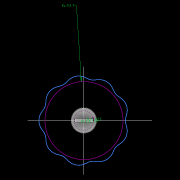
# Autodesk Inventor part: OuterRaceTool
Saved by Autodesk Inventor 2022.2 (Build 262287010, 287A)
## iProperties
Created: 2022-05-21
Part Number: OuterRaceTool
Material: Generic
Document SubType Name: Modeling
Designer: Árni Þór Þorgeirsson
Density: 1 g/cm^3
Appearance: Default
Author: Árni Þór Þorgeirsson
Autodesk Inventor part; units mm, degrees
ref_plane "YZ Plane" through (0, 0, 0) normal (1, 0, 0) x (0, 1, 0)
ref_plane "XZ Plane" through (0, 0, 0) normal (0, 1, 0) x (-1, 0, 0)
sketch "Sketch7" plane through (0, 0, 0) normal (0, 1, 0) x (-1, 0, 0)
  line L0 (0, 0) -> (0, 15.7673)
  line L1 (0, 0) -> (-13.3368, 0) construction
  line L2 (0, 15.7673) -> (-13.3368, 0) construction
  line L3 (0, 15.7673) -> (-18.6413, 0) construction
  line L4 (0, 15.7673) -> (-12.4569, -5.231) construction
  line L5 (0, 0) -> (0, -15.7673)
  line L6 (0, -15.7673) -> (-13.3368, 0) construction
  line L7 (0, -15.7673) -> (-18.6413, 0) construction
  line L8 (0, -15.7673) -> (-12.4569, 5.231) construction
  line L9 (-12.4569, 5.231) -> (-18.6413, 0) construction
  line L10 (-9.3537, 0) -> (-18.5948, -7.8164) construction
  line L11 (-9.3537, 0) -> (-18.0926, 7.3915) construction
  line L12 (0, -29.7093) -> (0, 66.7435) projected
  line L13 (-53.5, -5.9919) -> (-53.5, 6.008)
  line L14 (17.5786, 0) -> (-94.9714, 0) projected
  line L15 (-15.989, 2.2434) -> (-10.6846, -2.2434) construction
  line L16 (-10.6846, 2.2434) -> (-15.989, -2.2434) construction
  line L17 (-26.151, -15.9303) -> (-40.3783, -15.9303) construction
  line L18 (-40.3783, -15.9303) -> (-40.3783, -12.7539) construction
  line L19 (-40.3783, -12.7539) -> (-26.151, -12.7539) construction
  line L20 (-26.151, -12.7539) -> (-26.151, -15.9303) construction
  point P0 (-53.5, 0)
  dimension "Roller_Side_difference" = -0.0003
  dimension "d90" = 15.7673
  dimension "d201" = 53.5
  dimension "d343" = 99.548
  dimension "d344" = 99.549
  dimension "d367" = 8.1
  constraints: 28 end point, 9 point on line, 3 midpoint, 3 vertical, 2 horizontal, 2 parallel, 2 perpendicular, 1 collinear, 1 symmetric about line, 2 other
  measures "d90" distance of L0.start L0.end
  measures "d201" distance between parallel lines of L5 L13
  measures "d343" angle of L10 L8
  measures "d344" angle of L7 L10
  measures "d367" distance of L3.end L8.end
sketch "Sketch1" plane through (0, 0, 0) normal (0, 0, 1) x (1, 0, 0)
  circle A0 centre (0, 0) radius 13.3368 construction
  line L0 (0, 0) -> (13.3368, 0)
  line L1 (0, 0) -> (13.3368, 4.025)
  line L2 (13.3368, 0) -> (13.3368, 4.025)
  circle A1 centre (0, 0) radius 53.5
  point P0 (56.8, 0)
  dimension "d56" = 13.3368
  dimension "d57" = 4.025
  dimension "d400" = 53.5
  dimension "d495" = 2.5
  dimension "d496" = 8
  dimension "d531" = 5.5
  dimension "d532" = 5.5
  dimension "d533" = 5.5
  dimension "d537" = 24.5
  dimension "d538" = 3
  dimension "d543" = 5.5
  dimension "d549" = 3
  dimension "d550" = 3
  dimension "d567" = 5.5
  dimension "d568" = 5.5
  constraints: 1 other
sketch "Roller1" plane through (0, 0, 0) normal (0, 1, 0) x (-1, 0, 0)
  line L0 (0, 15.7673) -> (-12.4569, -5.231) construction
  line L1 (0, 15.7673) -> (-18.6413, 0) construction
  line L2 (-9.3537, 0) -> (-18.0926, 7.3915) construction
  line L3 (0, -15.7673) -> (-18.6413, 0) construction
  line L4 (-9.4248, -0.0708) -> (-12.4245, -5.1274)
  line L5 (-12.4245, -5.1274) -> (-18.5445, 0.0491)
  line L6 (-18.5445, 0.0491) -> (-14.0556, 3.846)
  line L7 (-14.0556, 3.846) -> (-9.4248, -0.0708)
  line L8 (-11.7456, 1.8921) -> (-15.4898, -2.5346)
  line L9 (-10.9821, 1.2463) -> (-14.7263, -3.1804)
  point P0 (0, 0)
  point P1 (-15.4845, -2.5391)
  dimension "d345" = 0.025
  dimension "d346" = 0.025
  dimension "d347" = 0.1
  dimension "d348" = 0.1
  dimension "d349" = 99.549
  dimension "d350" = 99.548
  dimension "d357" = 1
  dimension "d369" = 4.0148
  constraints: 12 end point, 5 parallel, 4 point on line, 1 midpoint, 1 perpendicular
  measures "d345" distance between parallel lines of L0 L4
  measures "d346" distance between parallel lines of L1 L6
  measures "d347" distance between parallel lines of L3 L5
  measures "d348" distance between parallel lines of L2 L7
  measures "d349" angle of L6 L7
  measures "d350" angle of L4 L7
  measures "d357" distance between parallel lines of L8 L9
  measures "d369" distance from line of L4.end L8
sketch "Roller2" plane through (0, 0, 0) normal (0, 1, 0) x (-1, 0, 0)
  line L0 (0, -15.7673) -> (-12.4569, 5.231) construction
  line L1 (-9.3537, 0) -> (-18.5948, -7.8164) construction
  line L2 (0, -15.7673) -> (-18.6413, 0) construction
  line L3 (0, 15.7673) -> (-18.6413, 0) construction
  line L4 (-12.4245, 5.1274) -> (-9.4248, 0.0708)
  line L5 (-9.4248, 0.0708) -> (-14.0556, -3.846)
  line L6 (-14.0556, -3.846) -> (-18.5445, -0.0491)
  line L7 (-18.5445, -0.0491) -> (-12.4245, 5.1274)
  line L8 (-15.4845, 2.5391) -> (-11.7403, -1.8876)
  line L9 (-14.721, 3.1849) -> (-10.9767, -1.2418)
  point P0 (0, 0)
  dimension "d351" = 0.025
  dimension "d352" = 0.025
  dimension "d354" = 0.1
  dimension "d355" = 99.548
  dimension "d356" = 99.549
  dimension "d370" = 0.1
  dimension "d371" = 1
  constraints: 12 end point, 5 parallel, 3 point on line, 1 midpoint, 1 perpendicular
  measures "d351" distance between parallel lines of L0 L4
  measures "d352" distance between parallel lines of L2 L6
  measures "d354" distance between parallel lines of L1 L5
  measures "d355" angle of L5 L4
  measures "d356" angle of L6 L5
  measures "d370" distance from line of L3 L8.start
  measures "d371" distance between parallel lines of L9 L8
sketch "Sketch22" plane through (0, 0, 0) normal (0, 1, 0) x (-1, 0, 0)
  line L0 (-31.756, 8.0215) -> (-17.5287, 8.0215) construction
  line L1 (-17.5287, 8.0215) -> (-17.5287, 4.8451) construction
  line L2 (-17.5287, 4.8451) -> (-31.756, 4.8451) construction
  line L3 (-31.756, 4.8451) -> (-31.756, 8.0215) construction
  point P0 (0, 0)
  dimension "Roller_Side_difference" = -0.0003
  constraints: 2 other
sketch "Sketch2" plane through (0, 0, 0) normal (0, 1, 0) x (-1, 0, 0)
  line L0 (0, 0) -> (0, 13.3368) construction
  line L1 (0, 0) -> (-13.3368, 0) projected
  line L2 (0, 0) -> (0, -13.3368)
  line L3 (0, -13.3368) -> (-13.3368, 0) construction
  line L4 (0, 13.3368) -> (-13.3368, 0) construction
  line L5 (-78.8928, 52.9645) -> (0, 13.3368) construction
  line L6 (-34.8011, 15.91) -> (0, 13.3368) construction
  line L7 (-34.8011, 15.91) -> (0, -13.3368) construction
  line L8 (-48.3339, 16.9106) -> (0, -13.3368) construction
  point P0 (-17.4708, -4.134)
  constraints: 16 end point, 3 point on line, 1 perpendicular, 1 symmetric about line, 1 vertical
sketch "Sketch23" plane through (0, 0, 0) normal (0, 1, 0) x (-1, 0, 0)
  line L0 (0, -15.7673) -> (-12.4569, 5.231) construction
  line L1 (0, -15.7673) -> (-18.6413, 0) construction
  line L2 (0, 15.7673) -> (-12.4569, -5.231) construction
  line L3 (-12.4569, 5.231) -> (-18.6413, 0) construction
  line L4 (0, 15.7673) -> (-18.6413, 0) construction
  line L5 (-12.4569, 5.231) -> (-12.4569, -5.231) construction
  line L6 (17.5786, 0) -> (-94.9714, 0) projected
  line L7 (-11.4508, 3.731) -> (-9.2677, 0.051)
  line L8 (-9.2677, -0.051) -> (-11.4508, -3.731)
  line L9 (-14.3852, 3.731) -> (-18.7059, 0.0764)
  line L10 (-18.7059, -0.0764) -> (-14.3852, -3.731)
  arc A0 (-18.7059, 0.0764) -> (-18.7059, -0.0764) centre (-18.6413, 0) ccw
  arc A1 (-9.2677, -0.051) -> (-9.2677, 0.051) centre (-9.3537, 0) ccw
  line L11 (-11.4508, 3.731) -> (-11.4508, 5.231)
  line L12 (-11.4508, 5.231) -> (-1, 5.231)
  line L13 (-1, 5.231) -> (-1, -5.231)
  line L14 (-1, -5.231) -> (-11.4508, -5.231)
  line L15 (-11.4508, -5.231) -> (-11.4508, -3.731)
  line L16 (-14.3852, 3.731) -> (-14.3852, 5.231)
  line L17 (-14.3852, 5.231) -> (-53.5, 5.231)
  line L18 (-53.5, 5.231) -> (-53.5, -5.231)
  line L19 (-14.3852, -3.731) -> (-14.3852, -5.231)
  line L20 (-14.3852, -5.231) -> (-53.5, -5.231)
  line L21 (-12.4569, 5.231) -> (-12.4569, 5.231)
  line L22 (-12.4569, -5.231) -> (-12.4569, -5.231)
  line L23 (0, -29.7093) -> (0, 66.7435) projected
  line L24 (-18.7962, 0) -> (-53.5, 0)
  point P0 (0, 0)
  point P1 (-9.2374, 0)
  point P2 (-18.7413, 0)
  point P3 (-53.5, 0)
  dimension "d378" = 90
  dimension "d379" = 0.1
  dimension "d380" = 0.1
  dimension "d381" = 0.1
  dimension "d382" = 0.1
  dimension "d383" = 0.1
  dimension "d384" = 10.4619
  dimension "d385" = 0
  dimension "d386" = 0
  dimension "d391" = 1
  dimension "d392" = 53.5
  dimension "d393" = 1.5
  dimension "d394" = 1.5
  dimension "d395" = 1.5
  dimension "d396" = 1.5
  constraints: 36 end point, 10 point on line, 9 vertical, 4 horizontal, 4 parallel, 4 point on circle, 4 tangent, 2 centre point, 1 equal radius, 1 midpoint
  measures "d378" angle of L6 L5
  measures "d379" radius of A0
  measures "d380" distance between parallel lines of L9 L4
  measures "d381" distance between parallel lines of L10 L1
  measures "d382" distance between parallel lines of L0 L7
  measures "d383" distance between parallel lines of L2 L8
  measures "d384" distance of L0.end L2.end
  measures "d385" distance of L2.end L22.end
  measures "d386" distance of L0.end L21.end
  measures "d391" distance between parallel lines of L23 L13
  measures "d392" distance between parallel lines of L18 L23
  measures "d393" distance of L9.start L16.end
  measures "d394" distance of L7.start L11.end
  measures "d395" distance of L14.end L8.end
  measures "d396" distance of L10.end L19.end
sketch "Sketch44" plane through (0, 0, 0) normal (0, 1, 0) x (-1, 0, 0)
  line L0 (-18.7962, 0) -> (3.1509, -18.5634)
  line L1 (17.5786, 0) -> (-94.9714, 0) projected
  line L2 (-11.4508, 5.231) -> (-1, 5.231) projected
  line L3 (-14.3852, 5.231) -> (-53.5, 5.231) projected
  line L4 (0, 0) -> (0, 15.7673) projected
  line L5 (0, 0) -> (0, -15.8983)
  line L6 (-25.707, -7.6404) -> (3.3976, -7.6404)
  line L7 (-18.6413, 0) -> (0, -15.7673)
  point P0 (-3.6044, 0)
  point P1 (-9.6083, -7.6404)
  point P2 (0, -7.6404)
  dimension "d615" = 0.1
  constraints: 8 end point, 4 point on line, 2 horizontal, 1 parallel, 1 other
  measures "d615" distance between parallel lines of L0 L7
revolve "Revolution17" add sketch "Sketch44" angle 360 about axis through (0, 0, 0) along (0, 0, 1) contours L1 L5 L6 L7
sketch "Sketch45" plane through (0, 0, 0) normal (0, 0, 1) x (1, 0, 0)
  line L0 (-12.5, 2.5) -> (12.5, 2.5)
  line L1 (12.5, 2.5) -> (12.5, -2.5)
  line L2 (12.5, -2.5) -> (-12.5, -2.5)
  line L3 (-12.5, -2.5) -> (-12.5, 2.5)
  line L4 (-12.5, 2.5) -> (12.5, -2.5) construction
  line L5 (12.5, 2.5) -> (-12.5, -2.5) construction
  point P0 (0, 0)
  dimension "d617" = 25
  dimension "d618" = 5
  constraints: 12 end point, 2 midpoint, 2 parallel, 1 horizontal, 1 perpendicular
  measures "d617" distance of L1.end L2.end
  measures "d618" distance of L0.end L1.end
extrude "Extrusion39" add sketch "Sketch45" along normal blind 25
fillet "Fillet4" radius 10 2 edges at (-12.5, 0, 25) (12.5, 0, 25)
fillet "Fillet5" radius 0.5 1 edges at (-18.6413, 0, 0)
sketch "Sketch40" plane through (0, 0, -5.231) normal (0, 0, -1) x (-1, 0, 0)
  circle A0 centre (53.5, 0) radius 2.75 projected
  circle A1 centre (0, 0) radius 53.5 projected
  point P0 (53.4293, 2.7491)
  point P1 (53.4293, -2.7491)
  dimension "d585" = 8
  dimension "d587" = 1.75
  dimension "d589" = 3
  dimension "d592" = 2
  dimension "d593" = 12
  dimension "d594" = 12
  dimension "d611" = 360
  constraints: 18 point on circle, 10 centre point, 8 end point, 2 midpoint, 1 horizontal alignment, 1 vertical, 29 other
  measures "d589" diameter of A1
equation "\"Roller_Side_difference\" = -0.001568deg"
equation "\"Cycloid_Top_Plate_Fasner_Inner\" = 61.25"
equation "\"Cycloid_Top_Plate_Fasner_Outer\" = 85.75"
equation "\"Roller_Hole_Radius\" = 1"
equation "\"Distance_To_Bearing\" = 20.65135"
equation "\"d514\" = 0.2"
body "Solid1"
body "Solid5"
body "Solid6"
